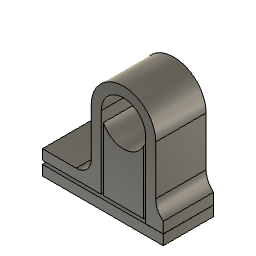
floorcowl_bottomfloor_edge v14 (Autodesk Fusion 360 design; units mm, degrees)
Autodesk Fusion 360 part; units mm, degrees
sketch "Sketch2" plane through (0, 0, 0) normal (0, 1, 0) x (1, 0, 0)
  circle A0 centre (0, 0) radius 9.525 construction
  circle A1 centre (0, 0) radius 11.176 construction
  line L0 (0, 0) -> (0, -11.176)
  line L1 (0, 0) -> (16.256, 0) construction
  line L2 (0, 0) -> (0, 36.576) construction
  arc A2 (-16.256, 0) -> (16.256, 0) centre (0, 0) ccw
  line L3 (0, 0) -> (-16.256, 0) construction
  line L4 (0, 0) -> (16.256, 0) construction
  line L5 (0, 36.576) -> (11.176, 36.576) construction
  line L6 (0, 36.576) -> (11.176, 36.576) construction
  line L7 (11.176, 36.576) -> (11.176, 38.3286) construction
  line L8 (11.176, 38.3286) -> (0, 38.3286) construction
  line L9 (0, 38.3286) -> (0, 36.576) construction
  line L10 (0, 36.576) -> (-25.4, 36.576) construction
  line L11 (-25.4, 36.576) -> (-25.4, 38.3286) construction
  line L12 (-25.4, 38.3286) -> (0, 38.3286) construction
  line L13 (16.256, 0) -> (11.176, 0)
  line L14 (11.176, 0) -> (11.176, 38.3286)
  line L15 (11.176, 38.3286) -> (16.256, 38.3286)
  line L16 (16.256, 38.3286) -> (16.256, 0)
  line L17 (16.256, 38.3286) -> (-40.894, 38.3286)
  line L18 (-40.894, 38.3286) -> (-40.894, 43.4086)
  line L19 (-40.894, 43.4086) -> (16.256, 43.4086)
  line L20 (16.256, 43.4086) -> (16.256, 38.3286)
  line L21 (-16.256, 0) -> (-11.176, 0)
  line L22 (-11.176, 0) -> (-11.176, 36.576)
  line L23 (-11.176, 36.576) -> (-16.256, 36.576)
  line L24 (-16.256, 36.576) -> (-16.256, 0)
  line L25 (-40.894, 38.3286) -> (-40.894, 25.6286)
  line L26 (-16.256, 36.576) -> (-40.894, 36.576)
  line L27 (-40.894, 36.576) -> (-40.894, 31.496) construction
  line L28 (-40.894, 31.496) -> (-16.256, 31.496)
  line L29 (-16.256, 31.496) -> (-16.256, 36.576) construction
  arc A3 (10.1289, 4.7232) -> (0, 11.176) centre (0, 0) ccw
  line L30 (0, 0) -> (10.1289, 4.7232) construction
  line L31 (0, 0) -> (0, 11.176) construction
  line L32 (10.1289, 4.7232) -> (10.1289, 36.576)
  line L33 (10.1289, 36.576) -> (0, 36.576)
  line L34 (-10.1289, 4.7232) -> (-10.1289, 36.576)
  arc A4 (0, 11.176) -> (-10.1289, 4.7232) centre (0, 0) ccw
  line L35 (0, 36.576) -> (-10.1289, 36.576)
  arc A5 (-11.176, 0) -> (11.176, 0) centre (0, 0) ccw
  line L36 (-10.1289, 4.7232) -> (-16.256, 4.7232) construction
  line L37 (11.176, 36.576) -> (11.176, 0)
  line L38 (11.176, 36.576) -> (16.256, 36.576)
  line L39 (16.256, 36.576) -> (20.066, 36.576)
  line L40 (16.256, 38.3286) -> (20.066, 38.3286)
  line L41 (20.066, 36.576) -> (20.066, 32.766)
  line L42 (20.066, 32.766) -> (16.256, 32.766)
  line L43 (16.256, 32.766) -> (16.256, 0)
  line L44 (20.066, 38.3286) -> (20.066, 43.4086)
  line L45 (16.256, 43.4086) -> (20.066, 43.4086)
  line L46 (20.066, 36.576) -> (20.066, 38.2778)
  line L47 (11.176, 36.576) -> (20.066, 36.576)
  line L48 (20.066, 36.576) -> (20.066, 38.2778)
  line L49 (20.066, 38.2778) -> (11.176, 38.2778)
  line L50 (11.176, 38.2778) -> (11.176, 36.576)
  dimension "d18" = 19.05
  dimension "d19" = 22.352
  dimension "d20" = 16.256
  dimension "d21" = 36.576
  dimension "d22" = 180
  dimension "d23" = 11.176
  dimension "d24" = 11.176
  dimension "d25" = 1.7526
  dimension "d26" = 5.08
  dimension "d27" = 38.3286
  dimension "d28" = 1.7526
  dimension "d29" = 25.4
  dimension "d30" = 5.08
  dimension "d31" = 57.15
  dimension "d32" = 5.08
  dimension "d33" = 36.576
  dimension "d35" = 12.7
  dimension "d36" = 24.638
  dimension "d37" = 5.08
  dimension "d38" = 11.176
  dimension "d39" = 65
  dimension "d41" = 11.176
  dimension "d83" = 36.576
  dimension "d84" = 3.81
  dimension "d85" = 3.81
  dimension "d86" = 3.81
  dimension "d87" = 5.08
  dimension "d100" = 1.7018
  constraint coincident A0.centre A1.centre
  constraint coincident A1 L0.end
  constraint vertical L0
  constraint perpendicular L0 L1
  constraint perpendicular L1 L2
  constraint perpendicular L2 L5
  constraint horizontal L6
  constraint vertical L7
  constraint horizontal L8
  constraint vertical L9
  constraint symmetric L2.end L9 L5.start
  constraint symmetric L8.end L9 L12.end
  constraint horizontal L13
  constraint vertical L14
  constraint horizontal L15
  constraint vertical L16
  constraint horizontal L12
  constraint horizontal L10
  constraint vertical L11
  constraint horizontal L17
  constraint vertical L18
  constraint horizontal L19
  constraint vertical L20
  constraint horizontal L21
  constraint vertical L22
  constraint horizontal L23
  constraint vertical L24
  constraint vertical L25
  constraint horizontal L26
  constraint vertical L27
  constraint horizontal L28
  constraint vertical L29
  constraint coincident L2 A3.end
  constraint vertical L32
  constraint symmetric L2 A3.start L34.start
  constraint symmetric L2 A3.end L31.end
  constraint symmetric L2 A3 A4
  constraint symmetric L2 L32.end L34.end
  constraint coincident L24 L36.end
  constraint perpendicular L24 L36
  constraint coincident L5 L32.end
  constraint horizontal L38
  constraint perpendicular L16 L39
  constraint perpendicular L20 L40
  constraint perpendicular L39 L41
  constraint coincident L16 L42.end
  constraint perpendicular L16 L42
  constraint perpendicular L40 L44
  constraint perpendicular L39 L46
  constraint horizontal L47
  constraint vertical L48
  constraint horizontal L49
  constraint vertical L50
  measures "d18" diameter of A0
  measures "d19" diameter of A1
  measures "d20" distance of A0.centre L1.end
  measures "d21" distance of A0.centre L2.end
  measures "d22" angle of L3 L4
  measures "d23" distance of L2.end L5.end
  measures "d24" distance of L2.end L5.end
  measures "d25" distance of L2.end L8.end
  measures "d26" distance of L1.end L13.end
  measures "d27" distance of L1.end L15.end
  measures "d28" distance of L10.end L11.end
  measures "d29" distance of L2.end L10.end
  measures "d30" distance of L15.end L19.end
  measures "d31" distance of L18.end L19.end
  measures "d32" distance of A2.start L21.end
  measures "d33" distance of A2.start L23.end
  measures "d35" distance of L17.end L25.end
  measures "d36" distance of L23.end L26.end
  measures "d37" distance of L23.end L28.end
  measures "d38" radius of A3
  measures "d39" angle of L30 L31
  measures "d41" radius of A5
  measures "d83" distance of L1.end L38.end
  measures "d84" distance of L38.end L39.end
  measures "d85" distance of L15.end L40.end
  measures "d86" distance of L39.end L41.end
  measures "d87" distance of L40.end L44.end
  measures "d100" distance of L39.end L46.end
extrude "Extrude1" add sketch "Sketch2" along normal blind 25.4 contours A2 L13 L21 A5 | L21 L22 L23 L24 | L24 L25 L26 L28 | L15 L17 L18 L19 L20 | L20 L40 L44 L45 | A3 L32 L33 L34 A4 L35 makes body 1 at (8.8196, 8.4667, 13.6555) makes body 2 at (-10.1289, 8.4667, -15.3408) makes body 3 at (-0.254, 8.4667, -38.3286)
extrude "Extrude2" add sketch "Sketch2" along normal blind 25.4 contours L13 L14 L16 L37 L38 L43 L47 | L16 L39 L41 L42 L47 bodies 1
extrude "Extrude3" add sketch "Sketch2" along normal blind 25.4 contours L14 L16 L38 L47 L49 L50 | L16 L39 L46 L47 L48 L49 bodies 1
sketch "Sketch6" plane through (-16.256, 0, 0) normal (-1, 0, 0) x (0, -1, 0)
  line L0 (0, -31.496) -> (0, 0)
  line L1 (0, 0) -> (-25.4, 0)
  line L2 (-25.4, 0) -> (-25.4, -31.496)
  line L3 (-25.4, -31.496) -> (0, -31.496)
  line L4 (0, -31.496) -> (0, -7.8994)
  line L5 (0, -7.8994) -> (-25.4, -7.8994)
  line L6 (-25.4, -7.8994) -> (-25.4, -31.496)
  line L7 (-12.7, -7.8994) -> (-12.7, -31.496)
  line L8 (-25.4, -16.2814) -> (0, -16.2814) construction
  line L9 (-25.4, -31.496) -> (0, -31.496)
  point P0 (-12.7, -16.2814)
  dimension "d54" = 23.5966
  dimension "d55" = 90
  dimension "d56" = 25.4
  dimension "d57" = 8.382
  constraint horizontal L3
  constraint vertical L4
  constraint horizontal L5
  constraint vertical L6
  constraint coincident L0 L4.end
  constraint coincident L2.end L3.start
  constraint midpoint L5 L7.start
  constraint coincident L6 L8.start
  constraint midpoint L8 P0
  measures "d54" distance of L2.end L5.end
  measures "d55" angle of L7 L8
  measures "d56" distance of L8.start L8.end
  measures "d57" distance of L5 L8
fillet "Fillet2" radius 10.16 1 edges at (16.256, 12.7, -32.766) on bodies 1
fillet "Fillet1" radius 7.62 1 edges at (-16.256, 12.7, -31.496) on bodies 1
sketch "Sketch7" plane through (0, 0, -43.4086) normal (0, 0, -1) x (1, 0, 0)
  line L0 (20.066, 0) -> (-40.894, 0)
  line L1 (-40.894, 0) -> (-40.894, -25.4)
  line L2 (-40.894, -25.4) -> (20.066, -25.4)
  line L3 (-40.894, 0) -> (-16.256, 0)
  line L4 (-16.256, 0) -> (-16.256, -25.4)
  line L5 (-16.256, -25.4) -> (-40.894, -25.4)
  line L6 (-40.894, -25.4) -> (-40.894, 0)
  line L7 (-28.575, 0) -> (-28.575, -25.4)
  line L8 (-40.894, -12.7) -> (-16.256, -12.7)
  line L9 (20.066, -25.4) -> (20.066, 0)
  line L10 (15.621, 0) -> (15.621, -25.4)
  line L11 (-16.256, -12.7) -> (20.066, -12.7)
  point P0 (-28.575, -6.35)
  point P1 (-28.575, -19.05)
  point P2 (15.621, -6.35)
  point P3 (15.621, -19.05)
  dimension "d75" = 24.638
  dimension "d76" = 25.4
  dimension "d77" = 6.35
  dimension "d92" = 8.89
  dimension "d93" = 6.35
  dimension "d94" = 6.35
  constraint horizontal L3
  constraint vertical L4
  constraint horizontal L5
  constraint vertical L6
  constraint coincident L0.end L1.start
  constraint midpoint L3 L7.start
  constraint midpoint L5 L7.end
  constraint midpoint L1 L8.start
  constraint midpoint L4 L8.end
  constraint coincident L7 P0
  constraint symmetric L8 P0 P1
  constraint coincident L0 L10.start
  constraint coincident L2 L10.end
  constraint perpendicular L2 L10
  constraint midpoint L9 L11.end
  constraint coincident L10 P2
  constraint coincident L10 P3
  measures "d75" distance of L0.end L3.end
  measures "d76" distance of L0.end L1.end
  measures "d77" distance of L3 P0
  measures "d93" distance of L10.end P3
  measures "d94" distance of L0 P2
hole "Hole2" at (-16.256, 12.7, -16.2814) direction (1, 0, 0) diameter 4.2418 depth 30 tip angle 180 bodies 1 2
thread "Thread2" "ISO Metric profile 5.0 M5x0.8 M5x0.8 6H" major diameter 5.12 minor diameter 4.234 pitch 0.8 angle 60 resizes the face on face at (-14.5627, 12.8057, -14.1631) on face at (3.3763, 12.9112, -14.171) on face at (12.032, 12.8057, -14.1631) on bodies 1 2
hole "Hole5" at (-28.575, 6.35, -43.4086) at (-28.575, 19.05, -43.4086) at (15.621, 6.35, -43.4086) at (15.621, 19.05, -43.4086) direction (0, 0, 1) diameter 2.8702 depth 11.1125 tip angle 180 bodies 3 1
equation "d20 = 0.44 in + 0.2 in"
equation "d21 = 1 in + 0.44 in"
equation "d27 = 1.44 in + 0.069 in"
equation "d95 = ( 7 / 16 ) * 1 in"
